Autodesk Inventor part; units mm, degrees
(part 4 of 9)
sketch "Sketch27" plane through (0, 0, 0) normal (1, 0, 0) x (0, 0, -1)
  circle A0 centre (0, 0) radius 14.2875
  circle A1 centre (-101.8395, -75.4579) radius 31.75
  line L0 (-136.8494, 13.4274) -> (-99.9912, -11.4177)
  line L1 (-99.9912, -11.4177) -> (-75.1461, 25.4405)
  line L2 (-75.1461, 25.4405) -> (-112.0043, 50.2856)
  line L3 (-112.0043, 50.2856) -> (-136.8494, 13.4274)
  line L4 (-136.8494, 13.4274) -> (-75.1461, 25.4405) construction
  line L5 (-99.9912, -11.4177) -> (-112.0043, 50.2856) construction
  circle A2 centre (-101.8395, -75.4579) radius 44.565
  circle A3 centre (0, 0) radius 15.915
  line L6 (-119.5903, -34.5807) -> (-6.3391, 14.598)
  line L7 (-67.9013, -104.3411) -> (12.12, -10.3147)
  circle A4 centre (0, 0) radius 47.752
  line L8 (-107.8805, 35.2378) -> (-5.6488, 47.4167)
  circle A5 centre (-105.9978, 19.434) radius 15.9156
  line L9 (-113.3646, 5.3259) -> (-22.1029, -42.3286)
  line L10 (-100.8674, 14.1953) -> (-107.9694, 12.3717)
  line L11 (-107.9694, 12.3717) -> (-113.0997, 17.6103)
  line L12 (-113.0997, 17.6103) -> (-111.1281, 24.6726)
  line L13 (-111.1281, 24.6726) -> (-104.0262, 26.4963)
  line L14 (-104.0262, 26.4963) -> (-98.8958, 21.2576)
  line L15 (-98.8958, 21.2576) -> (-100.8674, 14.1953)
  circle A6 centre (-105.9978, 19.434) radius 7.3323
  circle A7 centre (-101.8395, -75.4579) radius 9.5631
  circle A8 centre (-105.9978, 19.434) radius 9.5631
  circle A9 centre (-101.8395, -75.4579) radius 25.4
  circle A10 centre (-105.9978, 19.434) radius 25.4
  line L16 (-101.8395, -75.4579) -> (0, 0)
  circle A11 centre (0, 0) radius 50.8
  circle A12 centre (-105.9978, 19.434) radius 31.4309
  arc A13 (136.2027, -114.2876) -> (161.1415, 75.1415) centre (0, 0) ccw
  line L17 (0, 0) -> (136.2027, -114.2876)
  line L18 (0, 0) -> (173.2597, 0)
  circle A14 centre (33.8645, -135.5333) radius 88.9
  circle A15 centre (-76.4174, -178.6042) radius 25.4
  line L19 (-88.4199, -21.0451) -> (-93.4785, -9.396)
  circle A16 centre (-76.4174, -178.6042) radius 21.4859
  line L20 (-141.7593, -95.2683) -> (-95.6637, -188.1553)
  line L21 (-57.286, -74.4485) -> (-54.9371, -178.1175)
  line L22 (136.2027, -114.2876) -> (90.5518, -239.7125)
  circle A17 centre (31.6927, -141.5004) radius 88.9
  line L23 (-52.5492, -187.2916) -> (90.6599, -239.4154)
  line L24 (-105.9978, 19.434) -> (0, 0)
  line L25 (-76.4174, -204.0042) -> (-76.4174, -178.6042)
  line L26 (136.2027, -114.2876) -> (136.2027, -239.7125)
  line L27 (-58.8554, 19.434) -> (-105.9978, 19.434)
  circle A18 centre (-17.4502, -276.5193) radius 88.9
  line L28 (-501.4434, -455.6125) -> (248.5176, -455.6125)
  line L29 (-550.7161, -581.025) -> (328.0098, -581.025)
  circle A19 centre (-54.61, -366.7125) radius 88.9
  line L30 (-54.61, -280.9875) -> (-16.51, -280.9875)
  line L31 (-16.51, -280.9875) -> (-16.51, -363.5375)
  line L32 (-16.51, -363.5375) -> (-54.61, -363.5375)
  line L33 (-54.61, -363.5375) -> (-54.61, -280.9875)
  line L34 (-54.61, -322.2625) -> (-16.51, -322.2625)
  line L35 (-54.61, -366.7125) -> (-54.61, -277.8125)
  circle A20 centre (-16.51, -277.8125) radius 88.9
  line L36 (-16.51, -277.8125) -> (-16.51, -366.7125)
  circle A21 centre (-180.2765, -142.3655) radius 31.75
  circle A22 centre (-180.2765, -142.3655) radius 25.4
  circle A23 centre (-180.2765, -142.3655) radius 44.563
  circle A24 centre (-180.2765, -142.3655) radius 9.5631
  line L37 (-194.9575, -184.4408) -> (-91.0984, -220.6795)
  line L38 (-165.5955, -100.2902) -> (-61.7364, -136.5289)
  circle A25 centre (-76.4174, -178.6042) radius 44.563
  line L39 (-167.0299, -113.5109) -> (-119.1112, -9.1307)
  line L40 (-156.1209, -121.7605) -> (-135.7449, -104.3796)
  circle A26 centre (29.8359, -136.4768) radius 88.9
  line L41 (-116.4833, -117.4265) -> (-112.2994, -105.4355)
  line L42 (-85.3603, 16.259) -> (-85.3603, 6.734) projected
  arc A27 (-90.1228, 1.9715) -> (-85.3603, 6.734) centre (-90.1228, 6.734) ccw projected
  line L43 (-90.1228, 1.9715) -> (-121.8728, 1.9715) projected
  arc A28 (-126.6353, 6.734) -> (-121.8728, 1.9715) centre (-121.8728, 6.734) ccw projected
  line L44 (-126.6353, 6.734) -> (-126.6353, 16.259) projected
  line L45 (-126.6353, 16.259) -> (-132.3503, 16.259) projected
  arc A29 (-132.3503, 22.609) -> (-132.3503, 16.259) centre (-132.3503, 19.434) ccw projected
  line L46 (-132.3503, 22.609) -> (-126.6353, 22.609) projected
  line L47 (-126.6353, 22.609) -> (-126.6353, 32.134) projected
  arc A30 (-121.8728, 36.8965) -> (-126.6353, 32.134) centre (-121.8728, 32.134) ccw projected
  line L48 (-121.8728, 36.8965) -> (-90.1228, 36.8965) projected
  arc A31 (-85.3603, 32.134) -> (-90.1228, 36.8965) centre (-90.1228, 32.134) ccw projected
  line L49 (-85.3603, 32.134) -> (-85.3603, 22.609) projected
  line L50 (-85.3603, 22.609) -> (-79.6453, 22.609) projected
  arc A32 (-79.6453, 16.259) -> (-79.6453, 22.609) centre (-79.6453, 19.434) ccw projected
  line L51 (-79.6453, 16.259) -> (-85.3603, 16.259) projected
  circle A33 centre (-76.4174, -178.6042) radius 13.335 projected
  circle A34 centre (-187.1176, -166.8269) radius 2.4892 projected
  circle A35 centre (-174.2102, -166.8866) radius 2.4892 projected
  circle A36 centre (-167.2175, -120.5501) radius 2.4892 projected
  circle A37 centre (-180.1195, -116.9252) radius 2.4892 projected
  circle A38 centre (-193.0957, -120.1058) radius 2.4892 projected
  circle A39 centre (-186.8225, -117.6771) radius 2.4892 projected
  circle A40 centre (-173.4354, -117.9041) radius 2.4892 projected
  circle A41 centre (-168.1768, -164.3742) radius 2.4892 projected
  circle A42 centre (-180.6733, -167.7222) radius 2.4892 projected
  circle A43 centre (-193.0957, -164.2646) radius 2.4892 projected
  arc A44 (-177.4857, -133.2108) -> (-183.7867, -151.2692) centre (-180.6362, -142.24) ccw projected
  arc A45 (-183.3071, -151.4366) -> (-177.0061, -133.3781) centre (-180.1566, -142.4074) ccw projected
  circle A46 centre (-85.7798, -94.9817) radius 2.4892 projected
  circle A47 centre (-110.3931, -99.2933) radius 2.4892 projected
  circle A48 centre (-101.8395, -50.0579) radius 2.4892 projected
  circle A49 centre (-124.2369, -62.8574) radius 2.4892 projected
  circle A50 centre (-110.6604, -51.6228) radius 2.4892 projected
  circle A51 centre (-93.2858, -99.3592) radius 2.4892 projected
  circle A52 centre (-118.4334, -56.0666) radius 2.4892 projected
  circle A53 centre (-93.0185, -51.5569) radius 2.4892 projected
  circle A54 centre (-101.8395, -100.8579) radius 2.4892 projected
  circle A55 centre (-80.2428, -88.2574) radius 2.4892 projected
  arc A56 (-99.4903, -84.728) -> (-104.0551, -66.155) centre (-101.7058, -75.4251) ccw projected
  arc A57 (-99.6119, -84.758) -> (-99.4903, -84.728) centre (-101.8395, -75.4579) ccw projected
  arc A58 (-99.7334, -84.7881) -> (-99.6119, -84.758) centre (-101.9731, -75.491) ccw projected
  arc A59 (-99.8547, -84.8183) -> (-99.7334, -84.7881) centre (-102.1066, -75.5241) ccw projected
  arc A60 (-104.4917, -66.2632) -> (-99.8547, -84.8183) centre (-102.2399, -75.5574) ccw projected
  arc A61 (-104.3463, -66.227) -> (-104.4917, -66.2632) centre (-102.1066, -75.5241) ccw projected
  arc A62 (-104.2008, -66.1909) -> (-104.3463, -66.227) centre (-101.9731, -75.491) ccw projected
  arc A63 (-104.0551, -66.155) -> (-104.2008, -66.1909) centre (-101.8395, -75.4579) ccw projected
  circle A64 centre (239.2356, -31.496) radius 3.3782 projected
  circle A65 centre (223.7295, 90.3926) radius 3.3782 projected
  circle A66 centre (239.2356, 31.496) radius 3.3782 projected
  circle A67 centre (221.404, -95.9477) radius 3.3782 projected
  line L52 (-35.2916, -50.8) -> (42.0514, -50.8) projected
  arc A68 (74.705, -62.6849) -> (42.0514, -50.8) centre (42.0514, -101.6) ccw projected
  line L53 (74.705, -62.6849) -> (143.4787, -120.3929) projected
  arc A69 (143.8351, -124.9069) -> (143.4787, -120.3929) centre (141.4378, -122.8251) ccw projected
  arc A70 (141.8978, -127.1034) -> (143.8351, -124.9069) centre (0, 0) ccw projected
  arc A71 (141.8978, -127.1034) -> (141.494, -128.2246) centre (143.0803, -128.1626) ccw projected
  line L54 (141.6194, -131.4328) -> (141.494, -128.2246) projected
  arc A72 (141.6194, -131.4328) -> (142.123, -132.5318) centre (143.2057, -131.3708) ccw projected
  line L55 (142.123, -132.5318) -> (176.2311, -164.3381) projected
  arc A73 (176.2311, -164.3381) -> (194.6236, -163.2104) centre (184.8924, -155.0499) ccw projected
  arc A74 (194.6236, -163.2104) -> (235.5329, 95.0804) centre (0, 0) ccw projected
  arc A75 (235.5329, 95.0804) -> (218.389, 101.8364) centre (223.7562, 90.3263) ccw projected
  line L56 (218.389, 101.8364) -> (173.6183, 80.9596) projected
  arc A76 (152.1493, 76.2) -> (173.6183, 80.9596) centre (152.1493, 127) ccw projected
  line L57 (152.1493, 76.2) -> (-101.6, 76.2) projected
  line L58 (-101.6, 76.2) -> (-199.482, -21.682) projected
  line L59 (-199.482, -21.682) -> (-199.482, -255.599) projected
  line L60 (-199.482, -255.599) -> (-35.2916, -255.599) projected
  line L61 (-35.2916, -255.599) -> (-35.2916, -50.8) projected
  line L62 (149.831, -89.2272) -> (89.9434, -38.9755) projected
  arc A77 (88.9, -36.7379) -> (89.9434, -38.9755) centre (91.821, -36.7379) ccw projected
  line L63 (88.9, -36.7379) -> (88.9, -15.621) projected
  arc A78 (91.821, -12.7) -> (88.9, -15.621) centre (91.821, -15.621) ccw projected
  line L64 (91.821, -12.7) -> (174.1799, -12.7) projected
  arc A79 (177.0893, -15.8819) -> (174.1799, -12.7) centre (174.1799, -15.621) ccw projected
  arc A80 (154.2425, -88.4425) -> (177.0893, -15.8819) centre (0, 0) ccw projected
  arc A81 (149.831, -89.2272) -> (154.2425, -88.4425) centre (151.7086, -86.9895) ccw projected
  line L65 (88.9, -0.254) -> (88.9, 0.254) projected
  arc A82 (91.821, 3.175) -> (88.9, 0.254) centre (91.821, 0.254) ccw projected
  line L66 (91.821, 3.175) -> (174.4218, 3.175) projected
  arc A83 (177.3428, 0.254) -> (174.4218, 3.175) centre (174.4218, 0.254) ccw projected
  line L67 (177.3428, 0.254) -> (177.3428, -0.254) projected
  arc A84 (174.4218, -3.175) -> (177.3428, -0.254) centre (174.4218, -0.254) ccw projected
  line L68 (174.4218, -3.175) -> (91.821, -3.175) projected
  arc A85 (88.9, -0.254) -> (91.821, -3.175) centre (91.821, -0.254) ccw projected
  arc A86 (177.0893, 15.8819) -> (169.6939, 53.0738) centre (0, 0) ccw projected
  arc A87 (174.1799, 12.7) -> (177.0893, 15.8819) centre (174.1799, 15.621) ccw projected
  line L69 (174.1799, 12.7) -> (91.821, 12.7) projected
  arc A88 (88.9, 15.621) -> (91.821, 12.7) centre (91.821, 15.621) ccw projected
  line L70 (88.9, 15.621) -> (88.9, 17.1891) projected
  arc A89 (90.5865, 19.8364) -> (88.9, 17.1891) centre (91.821, 17.1891) ccw projected
  line L71 (90.5865, 19.8364) -> (165.6716, 54.8492) projected
  arc A90 (169.6939, 53.0738) -> (165.6716, 54.8492) centre (166.9061, 52.2019) ccw projected
  arc A91 (180.8991, -105.7674) -> (203.0448, 51.8076) centre (0, 0) ccw projected
  arc A92 (204.8485, 54.889) -> (203.0448, 51.8076) centre (205.5059, 52.4355) ccw projected
  line L72 (204.8485, 54.889) -> (206.0753, 55.2177) projected
  arc A93 (209.1938, 53.3924) -> (206.0753, 55.2177) centre (206.7327, 52.7643) ccw projected
  arc A94 (186.3731, -108.9857) -> (209.1938, 53.3924) centre (0, 0) ccw projected
  arc A95 (182.8723, -109.8807) -> (186.3731, -108.9857) centre (184.1805, -107.7035) ccw projected
  line L73 (182.8723, -109.8807) -> (181.7836, -109.2266) projected
  arc A96 (180.8991, -105.7674) -> (181.7836, -109.2266) centre (183.0918, -107.0494) ccw projected
  arc A97 (159.1231, -92.6879) -> (178.5072, 45.237) centre (0, 0) ccw projected
  arc A98 (180.312, 48.3145) -> (178.5072, 45.237) centre (180.9694, 45.861) ccw projected
  line L74 (180.312, 48.3145) -> (181.5388, 48.6432) projected
  arc A99 (184.6584, 46.8139) -> (181.5388, 48.6432) centre (182.1962, 46.1897) ccw projected
  arc A100 (164.6013, -95.8992) -> (184.6584, 46.8139) centre (0, 0) ccw projected
  arc A101 (161.0985, -96.7977) -> (164.6013, -95.8992) centre (162.4067, -94.6205) ccw projected
  line L75 (161.0985, -96.7977) -> (160.0098, -96.1436) projected
  arc A102 (159.1231, -92.6879) -> (160.0098, -96.1436) centre (161.3179, -93.9664) ccw projected
  line L76 (171.9854, -103.3393) -> (170.8967, -102.6851) projected
  arc A103 (170.0112, -99.2275) -> (170.8967, -102.6851) centre (172.2049, -100.5079) ccw projected
  arc A104 (170.0112, -99.2275) -> (190.7761, 48.5222) centre (0, 0) ccw projected
  arc A105 (192.5803, 51.6017) -> (190.7761, 48.5222) centre (193.2377, 49.1483) ccw projected
  line L77 (192.5803, 51.6017) -> (193.8071, 51.9305) projected
  arc A106 (196.9261, 50.1033) -> (193.8071, 51.9305) centre (194.4645, 49.477) ccw projected
  arc A107 (175.4872, -102.4426) -> (196.9261, 50.1033) centre (0, 0) ccw projected
  arc A108 (171.9854, -103.3393) -> (175.4872, -102.4426) centre (173.2936, -101.1621) ccw projected
  circle A109 centre (187.962, 68.4126) radius 2.5527 projected
  circle A110 centre (160.7915, -118.9794) radius 2.5527 projected
  circle A111 centre (0, 0) radius 13.335 projected
  line L78 (-177.4857, -133.2108) -> (-177.0061, -133.3781) projected
  line L79 (-183.3071, -151.4366) -> (-183.7867, -151.2692) projected
  point P0 (-35.56, -322.2625)
  dimension "d821" = 63.5
  dimension "d820" = 28.575
  dimension "d822" = 44.45
  dimension "d823" = 31.83
  dimension "d824" = 89.13
  dimension "d825" = 95.504
  dimension "d826" = 31.8313
  dimension "d827" = 12.7
  dimension "d828" = 19.1262
  dimension "d829" = 19.1262
  dimension "d830" = 50.8
  dimension "d831" = 50.8
  dimension "d832" = 107.7646
  dimension "d833" = 126.7485
  dimension "d834" = 101.6
  dimension "d835" = 127
  dimension "d836" = 40
  dimension "d837" = 177.8
  dimension "d838" = 50.8
  dimension "d839" = 12.7
  dimension "d840" = 6.35
  dimension "d841" = 106.233
  dimension "d842" = 152.4
  dimension "d843" = 279.1458
  dimension "d844" = 25
  dimension "d845" = 20
  dimension "d846" = 47.1424
  dimension "d847" = 42.9717
  dimension "d848" = 125.4125
  dimension "d849" = 656.1665
  dimension "d850" = 82.55
  dimension "d851" = 38.1
  dimension "d852" = 1.5989
  dimension "d853" = 35.56
  dimension "d854" = 215.9
  dimension "d855" = 215.9
  dimension "d856" = 26.7819
  dimension "d857" = 114.8539
  dimension "d858" = 109.9998
  dimension "d859" = 581.025
  dimension "d860" = 455.6125
  dimension "d861" = 12.7
  dimension "d862" = 89.1261
  constraints: 84 end point, 26 point on circle, 24 tangent, 23 centre point, 19 coincident, 9 midpoint, 7 perpendicular, 6 equal radius, 6 horizontal, 6 line through centre, 6 point on line, 4 parallel, 4 vertical, 3 concentric, 2 vertical alignment, 26 other
  measures "d820" diameter of A0
  measures "d822" distance of L0.end L1.end
  measures "d823" diameter of A3
  measures "d824" diameter of A2
  measures "d825" diameter of A4
  measures "d826" diameter of A5
  measures "d827" distance between parallel lines of L14 L11
  measures "d828" diameter of A7
  measures "d829" diameter of A8
  measures "d830" diameter of A9
  measures "d831" diameter of A10
  measures "d832" distance of A0.centre point (-105.998, 19.434)
  measures "d833" distance of point (0, 0) point (-101.84, -75.458)
  measures "d834" diameter of A11
  measures "d835" radial gap between concentric circles of A13 A11
  measures "d836" angle of L18 L17
  measures "d837" diameter of A14
  measures "d838" diameter of A15
  measures "d839" distance of L19.start L19.end
  measures "d840" distance of A17.centre A14.centre
  measures "d841" distance of point (-101.84, -75.458) A15.centre
  measures "d842" distance of L23.start L23.end
  measures "d843" vertical distance of L25.start A13.end
  measures "d845" angle of L26 L22
  measures "d846" distance of point (-105.998, 19.434) L27.start
  measures "d847" diameter of A16
  measures "d848" distance between parallel lines of L28 L29
  measures "d849" distance from line of A13.end L29
  measures "d850" distance of L33.start L30.start
  measures "d851" distance of L31.end L33.start
  measures "d852" distance of L36.start A18.centre
  measures "d853" horizontal distance of A11.centre point (-35.56, -322.262)
  measures "d854" distance from line of L28 L26.end
  measures "d855" distance from line of L28 L22.end
  measures "d856" distance of L40.start L40.end
  measures "d857" distance of L39.start L39.end
  measures "d858" distance of A21.centre L25.end
  measures "d859" distance from line of L29 point (0, 0)
  measures "d860" distance from line of L28 L17.start
  measures "d861" distance of L41.start L41.end
  measures "d862" diameter of A23
hole "Hole10" at (0, 19.434, 58.8554) direction (-1, 0, 0) diameter 4.9784 end through all clearance for "Flat Head Machine Screw (82)" size "#10" standard "Ansi Unified Screw Threads"
sketch "Sketch28" plane through (0, 0, 0) normal (1, 0, 0) x (0, 0, -1)
  line L0 (-85.3603, 16.259) -> (-85.3603, 6.734) projected
  arc A0 (-90.1228, 1.9715) -> (-85.3603, 6.734) centre (-90.1228, 6.734) ccw projected
  line L1 (-90.1228, 1.9715) -> (-121.8728, 1.9715) projected
  arc A1 (-126.6353, 6.734) -> (-121.8728, 1.9715) centre (-121.8728, 6.734) ccw projected
  line L2 (-126.6353, 6.734) -> (-126.6353, 16.259) projected
  line L3 (-126.6353, 16.259) -> (-132.3503, 16.259) projected
  arc A2 (-132.3503, 22.609) -> (-132.3503, 16.259) centre (-132.3503, 19.434) ccw projected
  line L4 (-132.3503, 22.609) -> (-126.6353, 22.609) projected
  line L5 (-126.6353, 22.609) -> (-126.6353, 32.134) projected
  arc A3 (-121.8728, 36.8965) -> (-126.6353, 32.134) centre (-121.8728, 32.134) ccw projected
  line L6 (-121.8728, 36.8965) -> (-90.1228, 36.8965) projected
  arc A4 (-85.3603, 32.134) -> (-90.1228, 36.8965) centre (-90.1228, 32.134) ccw projected
  line L7 (-85.3603, 32.134) -> (-85.3603, 22.609) projected
  line L8 (-85.3603, 22.609) -> (-79.6453, 22.609) projected
  arc A5 (-79.6453, 16.259) -> (-79.6453, 22.609) centre (-79.6453, 19.434) ccw projected
  line L9 (-79.6453, 16.259) -> (-85.3603, 16.259) projected
  circle A6 centre (-187.1176, -166.8269) radius 2.4892 projected
  circle A7 centre (-174.2102, -166.8866) radius 2.4892 projected
  circle A8 centre (-167.2175, -120.5501) radius 2.4892 projected
  circle A9 centre (-180.1195, -116.9252) radius 2.4892 projected
  circle A10 centre (-193.0957, -120.1058) radius 2.4892 projected
  circle A11 centre (-186.8225, -117.6771) radius 2.4892 projected
  circle A12 centre (-173.4354, -117.9041) radius 2.4892 projected
  circle A13 centre (-168.1768, -164.3742) radius 2.4892 projected
  circle A14 centre (-180.6733, -167.7222) radius 2.4892 projected
  circle A15 centre (-193.0957, -164.2646) radius 2.4892 projected
  circle A16 centre (0, 0) radius 13.335 projected
  circle A17 centre (160.7915, -118.9794) radius 2.5527 projected
  line L10 (182.8723, -109.8807) -> (181.7836, -109.2266) projected
  arc A18 (170.0112, -99.2275) -> (190.7761, 48.5222) centre (0, 0) ccw projected
  line L11 (204.8485, 54.889) -> (206.0753, 55.2177) projected
  arc A19 (175.4872, -102.4426) -> (196.9261, 50.1033) centre (0, 0) ccw projected
  arc A20 (159.1231, -92.6879) -> (178.5072, 45.237) centre (0, 0) ccw projected
  line L12 (180.312, 48.3145) -> (181.5388, 48.6432) projected
  arc A21 (164.6013, -95.8992) -> (184.6584, 46.8139) centre (0, 0) ccw projected
  line L13 (161.0985, -96.7977) -> (160.0098, -96.1436) projected
  arc A22 (180.8991, -105.7674) -> (203.0448, 51.8076) centre (0, 0) ccw projected
  line L14 (192.5803, 51.6017) -> (193.8071, 51.9305) projected
  arc A23 (186.3731, -108.9857) -> (209.1938, 53.3924) centre (0, 0) ccw projected
  line L15 (171.9854, -103.3393) -> (170.8967, -102.6851) projected
  circle A24 centre (239.2356, -31.496) radius 3.3782 projected
  circle A25 centre (223.7295, 90.3926) radius 3.3782 projected
  circle A26 centre (239.2356, 31.496) radius 3.3782 projected
  circle A27 centre (221.404, -95.9477) radius 3.3782 projected
  line L16 (-35.2916, -50.8) -> (42.0514, -50.8) projected
  arc A28 (74.705, -62.6849) -> (42.0514, -50.8) centre (42.0514, -101.6) ccw projected
  line L17 (74.705, -62.6849) -> (143.4787, -120.3929) projected
  arc A29 (143.8351, -124.9069) -> (143.4787, -120.3929) centre (141.4378, -122.8251) ccw projected
  arc A30 (141.8978, -127.1034) -> (143.8351, -124.9069) centre (0, 0) ccw projected
  arc A31 (141.8978, -127.1034) -> (141.494, -128.2246) centre (143.0803, -128.1626) ccw projected
  line L18 (141.6194, -131.4328) -> (141.494, -128.2246) projected
  arc A32 (141.6194, -131.4328) -> (142.123, -132.5318) centre (143.2057, -131.3708) ccw projected
  line L19 (142.123, -132.5318) -> (176.2311, -164.3381) projected
  arc A33 (176.2311, -164.3381) -> (194.6236, -163.2104) centre (184.8924, -155.0499) ccw projected
  arc A34 (194.6236, -163.2104) -> (235.5329, 95.0804) centre (0, 0) ccw projected
  arc A35 (235.5329, 95.0804) -> (218.389, 101.8364) centre (223.7562, 90.3263) ccw projected
  line L20 (218.389, 101.8364) -> (173.6183, 80.9596) projected
  arc A36 (152.1493, 76.2) -> (173.6183, 80.9596) centre (152.1493, 127) ccw projected
  line L21 (152.1493, 76.2) -> (-101.6, 76.2) projected
  line L22 (-101.6, 76.2) -> (-199.482, -21.682) projected
  line L23 (-199.482, -21.682) -> (-199.482, -255.599) projected
  line L24 (-199.482, -255.599) -> (-35.2916, -255.599) projected
  line L25 (-35.2916, -255.599) -> (-35.2916, -50.8) projected
  line L26 (149.831, -89.2272) -> (89.9434, -38.9755) projected
  line L27 (88.9, -36.7379) -> (88.9, -15.621) projected
  line L28 (91.821, -12.7) -> (174.1799, -12.7) projected
  arc A37 (154.2425, -88.4425) -> (177.0893, -15.8819) centre (0, 0) ccw projected
  line L29 (88.9, -0.254) -> (88.9, 0.254) projected
  line L30 (91.821, 3.175) -> (174.4218, 3.175) projected
  line L31 (177.3428, 0.254) -> (177.3428, -0.254) projected
  line L32 (174.4218, -3.175) -> (91.821, -3.175) projected
  arc A38 (177.0893, 15.8819) -> (169.6939, 53.0738) centre (0, 0) ccw projected
  line L33 (174.1799, 12.7) -> (91.821, 12.7) projected
  line L34 (88.9, 15.621) -> (88.9, 17.1891) projected
  line L35 (90.5865, 19.8364) -> (165.6716, 54.8492) projected
  circle A39 centre (-80.2428, -88.2574) radius 2.4892 projected
  circle A40 centre (-101.8395, -100.8579) radius 2.4892 projected
  circle A41 centre (-93.0185, -51.5569) radius 2.4892 projected
  circle A42 centre (-93.2858, -99.3592) radius 2.4892 projected
  circle A43 centre (-110.6604, -51.6228) radius 2.4892 projected
  circle A44 centre (-124.2369, -62.8574) radius 2.4892 projected
  circle A45 centre (-101.8395, -50.0579) radius 2.4892 projected
  circle A46 centre (-110.3931, -99.2933) radius 2.4892 projected
  circle A47 centre (-85.7798, -94.9817) radius 2.4892 projected
  line L36 (-121.8728, 6.734) -> (-90.1228, 6.734)
  line L37 (-90.1228, 6.734) -> (-90.1228, 32.134)
  line L38 (-90.1228, 32.134) -> (-121.8728, 32.134)
  line L39 (-121.8728, 32.134) -> (-121.8728, 6.734)
  line L40 (-121.8728, 6.734) -> (-90.1228, 32.134) construction
  line L41 (-90.1228, 6.734) -> (-121.8728, 32.134) construction
  line L42 (-131.3978, 57.3308) -> (-80.5978, 57.3308)
  line L43 (-105.9978, 19.434) -> (-105.9978, 57.3308)
  line L44 (-105.9978, -16.3292) -> (-105.9978, 19.434)
  line L45 (-112.3478, -16.3292) -> (-99.6478, -16.3292)
  circle A48 centre (-112.3478, -16.3292) radius 2.5527
  circle A49 centre (-99.6478, -16.3292) radius 2.5527
  circle A50 centre (-80.5978, 57.3308) radius 2.5527
  circle A51 centre (-131.3978, 57.3308) radius 2.5527
  line L46 (-112.3478, -13.7765) -> (-99.6478, -13.7765)
  line L47 (-99.6478, -18.8819) -> (-112.3478, -18.8819)
  line L48 (-131.3978, 59.8835) -> (-80.5978, 59.8835)
  line L49 (-80.5978, 54.7781) -> (-131.3978, 54.7781)
  arc A52 (174.1799, 12.7) -> (177.0893, 15.8819) centre (174.1799, 15.621) ccw projected
  arc A53 (88.9, 15.621) -> (91.821, 12.7) centre (91.821, 15.621) ccw projected
  arc A54 (90.5865, 19.8364) -> (88.9, 17.1891) centre (91.821, 17.1891) ccw projected
  arc A55 (169.6939, 53.0738) -> (165.6716, 54.8492) centre (166.9061, 52.2019) ccw projected
  arc A56 (91.821, 3.175) -> (88.9, 0.254) centre (91.821, 0.254) ccw projected
  arc A57 (177.3428, 0.254) -> (174.4218, 3.175) centre (174.4218, 0.254) ccw projected
  arc A58 (174.4218, -3.175) -> (177.3428, -0.254) centre (174.4218, -0.254) ccw projected
  arc A59 (88.9, -0.254) -> (91.821, -3.175) centre (91.821, -0.254) ccw projected
  arc A60 (88.9, -36.7379) -> (89.9434, -38.9755) centre (91.821, -36.7379) ccw projected
  arc A61 (91.821, -12.7) -> (88.9, -15.621) centre (91.821, -15.621) ccw projected
  arc A62 (177.0893, -15.8819) -> (174.1799, -12.7) centre (174.1799, -15.621) ccw projected
  arc A63 (149.831, -89.2272) -> (154.2425, -88.4425) centre (151.7086, -86.9895) ccw projected
  arc A64 (170.0112, -99.2275) -> (170.8967, -102.6851) centre (172.2049, -100.5079) ccw projected
  arc A65 (192.5803, 51.6017) -> (190.7761, 48.5222) centre (193.2377, 49.1483) ccw projected
  arc A66 (196.9261, 50.1033) -> (193.8071, 51.9305) centre (194.4645, 49.477) ccw projected
  arc A67 (171.9854, -103.3393) -> (175.4872, -102.4426) centre (173.2936, -101.1621) ccw projected
  arc A68 (180.312, 48.3145) -> (178.5072, 45.237) centre (180.9694, 45.861) ccw projected
  arc A69 (184.6584, 46.8139) -> (181.5388, 48.6432) centre (182.1962, 46.1897) ccw projected
  arc A70 (161.0985, -96.7977) -> (164.6013, -95.8992) centre (162.4067, -94.6205) ccw projected
  arc A71 (159.1231, -92.6879) -> (160.0098, -96.1436) centre (161.3179, -93.9664) ccw projected
  arc A72 (204.8485, 54.889) -> (203.0448, 51.8076) centre (205.5059, 52.4355) ccw projected
  arc A73 (209.1938, 53.3924) -> (206.0753, 55.2177) centre (206.7327, 52.7643) ccw projected
  arc A74 (182.8723, -109.8807) -> (186.3731, -108.9857) centre (184.1805, -107.7035) ccw projected
  arc A75 (180.8991, -105.7674) -> (181.7836, -109.2266) centre (183.0918, -107.0494) ccw projected
  arc A76 (-99.6119, -84.758) -> (-99.4903, -84.728) centre (-101.8395, -75.4579) ccw projected
  arc A77 (-99.4903, -84.728) -> (-104.0551, -66.155) centre (-101.7058, -75.4251) ccw projected
  arc A78 (-99.7334, -84.7881) -> (-99.6119, -84.758) centre (-101.9731, -75.491) ccw projected
  arc A79 (-99.8547, -84.8183) -> (-99.7334, -84.7881) centre (-102.1066, -75.5241) ccw projected
  arc A80 (-104.4917, -66.2632) -> (-99.8547, -84.8183) centre (-102.2399, -75.5574) ccw projected
  arc A81 (-104.3463, -66.227) -> (-104.4917, -66.2632) centre (-102.1066, -75.5241) ccw projected
  arc A82 (-104.2008, -66.1909) -> (-104.3463, -66.227) centre (-101.9731, -75.491) ccw projected
  arc A83 (-104.0551, -66.155) -> (-104.2008, -66.1909) centre (-101.8395, -75.4579) ccw projected
  point P0 (-105.9978, 19.434)
  dimension "d478" = 50.8
  dimension "d479" = 12.7
  dimension "d480" = 5.1054
  dimension "d554" = 35.7632
  dimension "d555" = 37.8968
  constraints: 28 end point, 8 midpoint, 8 point on circle, 7 tangent, 6 coincident, 4 centre point, 4 horizontal, 3 equal radius, 2 parallel, 2 vertical, 1 perpendicular, 1 point on line
  measures "d478" distance of L42.end L42.start
  measures "d479" distance of L45.start L45.end
  measures "d480" diameter of A48
  measures "d554" distance from line of point (-105.998, 19.434) L45
  measures "d555" distance from line of L43.start L42
extrude "Extrusion17" cut sketch "Sketch28" against normal blind 25.4 contours L49 A51 L42 L22 | L22 L42 L43 L49 | L42 A51 L48 L22 | L22 L48 A50 L42 | L43 L42 A50 L49 | A51 | A50 | L45 A48 L46 L44 | L45 A49 L47 A48 | L44 L46 A49 L45 | A48 | A49
sketch "Sketch29" plane through (0, 0, 0) normal (1, 0, 0) x (0, 0, -1)
  arc A0 (194.6236, -163.2104) -> (235.5329, 95.0804) centre (0, 0) ccw projected
  line L0 (-199.482, -255.599) -> (-35.2916, -255.599) projected
  arc A1 (141.8978, -127.1034) -> (143.8351, -124.9069) centre (0, 0) ccw projected
  line L1 (74.705, -62.6849) -> (143.4787, -120.3929) projected
  line L2 (-35.2916, -255.599) -> (-35.2916, -50.8) projected
  line L3 (-35.2916, -255.599) -> (-35.2916, -230.199)
  line L4 (72.1517, -230.199) -> (-35.2916, -230.199)
  line L5 (142.123, -132.5318) -> (176.2311, -164.3381) projected
  line L6 (141.6194, -131.4328) -> (141.494, -128.2246) projected
  line L7 (-35.2916, -255.599) -> (149.8274, -255.599)
  line L8 (87.0583, -242.899) -> (183.6323, -242.899) construction
  circle A2 centre (145.0649, -113.4346) radius 6.35 construction
  line L9 (145.0649, -113.4346) -> (145.0649, -320.5339) construction
  line L10 (145.0649, -113.4346) -> (118.5854, -263.6072) construction
  line L11 (145.0649, -113.4346) -> (83.6885, -282.0649) construction
  line L12 (145.0649, -113.4346) -> (54.5486, -270.2133) construction
  arc A3 (154.2425, -88.4425) -> (177.0893, -15.8819) centre (0, 0) ccw construction
  line L13 (114.3, -157.1959) -> (114.3, -116.9566)
  arc A4 (176.2311, -164.3381) -> (194.6236, -163.2104) centre (184.8924, -155.0499) ccw construction
  line L14 (88.9, -36.7379) -> (88.9, -15.621) projected
  line L15 (149.8274, -255.599) -> (194.6236, -163.2104)
  line L16 (114.3, -157.1959) -> (72.1517, -230.199)
  line L17 (114.3, -116.9566) -> (179.2278, -123.3639)
  line L18 (179.2278, -123.3639) -> (194.6236, -163.2104)
  circle A5 centre (160.7915, -118.9794) radius 2.5527 projected
  arc A6 (143.8351, -124.9069) -> (143.4787, -120.3929) centre (141.4378, -122.8251) ccw projected
  point P0 (165.389, -138.7778)
  point P1 (102.5661, -230.199)
  point P2 (70.3186, -242.899)
  point P3 (97.9437, -242.899)
  point P4 (122.2368, -242.899)
  point P5 (145.0649, -242.899)
  point P6 (177.3458, -12.7)
  point P7 (152.4791, -91.4492)
  point P8 (184.8924, -167.7499)
  dimension "d495" = 25.4
  dimension "d497" = 12.7
  dimension "d498" = 12.7
  dimension "d499" = 10
  dimension "d501" = 20
  dimension "d502" = 30
  dimension "d507" = 4.7625
  dimension "d508" = 25.4
  dimension "d516" = 4.7625
  constraints: 26 end point, 9 point on line, 4 tangent, 2 coincident, 2 horizontal, 2 parallel, 1 centre point, 1 collinear, 1 point on circle, 1 vertical
  measures "d495" distance between parallel lines of L4 L7
  measures "d497" distance between parallel lines of L7 L8
  measures "d498" diameter of A2
  measures "d499" angle of L10 L9
  measures "d501" angle of L9 L11
  measures "d502" angle of L9 L12
  measures "d507" horizontal distance of L7.end point (145.065, -242.899)
  measures "d508" distance between parallel lines of L13 L14
  measures "d516" distance between parallel lines of L16 L12
extrude "Extrusion18" add sketch "Sketch29" against normal up to surface (3.175 mm away) contours L2 L4 L16 L13 L17 L18 L15 L7
fillet "Fillet7" radius 3.175 5 edges at (-1.5875, -157.1959, -114.3) (-1.5875, -230.199, -72.1517) (-1.5875, -230.199, 35.2916) (-1.5875, -50.8, 35.2916) (-1.5875, -163.2104, -194.6236)
hole "ChuteHoles" at (0, -242.899, -70.3186) at (0, -242.899, -97.9437) at (0, -242.899, -122.2368) at (0, -242.899, -145.0649) at (0, -113.4346, -145.0649) direction (-1, 0, 0) diameter 5.1054 end through all clearance for "Flat Head Machine Screw (82)" size "#10" standard "Ansi Unified Screw Threads"
sketch "Sketch32" plane through (0, 0, 0) normal (1, 0, 0) x (0, 0, -1)
  line L0 (152.1493, 76.2) -> (-101.6, 76.2) projected
  line L1 (-199.482, -255.599) -> (149.8274, -255.599) projected
  line L2 (-199.482, -21.682) -> (-199.482, -255.599) projected
  circle A0 centre (145.0649, -242.899) radius 2.5527 projected
  circle A1 centre (97.9437, -242.899) radius 2.5527 projected
  circle A2 centre (70.3186, -242.899) radius 2.5527 projected
  circle A3 centre (122.2368, -242.899) radius 2.5527 projected
  circle A4 centre (145.0649, -113.4346) radius 2.5527 projected
  line L3 (-35.2916, -227.024) -> (-35.2916, -53.975) projected
  arc A5 (-32.1166, -50.8) -> (-35.2916, -53.975) centre (-32.1166, -53.975) ccw projected
  line L4 (-32.1166, -50.8) -> (42.0514, -50.8) projected
  arc A6 (74.705, -62.6849) -> (42.0514, -50.8) centre (42.0514, -101.6) ccw projected
  line L5 (74.705, -62.6849) -> (142.7266, -119.7618) projected
  line L6 (114.3, -116.9566) -> (142.7266, -119.7618) projected
  line L7 (114.3, -156.3452) -> (114.3, -116.9566) projected
  arc A7 (113.8746, -157.9327) -> (114.3, -156.3452) centre (111.125, -156.3452) ccw projected
  line L8 (73.0682, -228.6115) -> (113.8746, -157.9327) projected
  arc A8 (70.3186, -230.199) -> (73.0682, -228.6115) centre (70.3186, -227.024) ccw projected
  line L9 (-32.1166, -230.199) -> (70.3186, -230.199) projected
  arc A9 (-35.2916, -227.024) -> (-32.1166, -230.199) centre (-32.1166, -227.024) ccw projected
  circle A10 centre (160.7915, -118.9794) radius 2.5527 projected
  circle A11 centre (0, 0) radius 13.335 projected
  circle A12 centre (187.962, 68.4126) radius 2.5527 projected
  line L10 (171.9854, -103.3393) -> (170.8967, -102.6851) projected
  arc A13 (170.0112, -99.2275) -> (170.8967, -102.6851) centre (172.2049, -100.5079) ccw projected
  arc A14 (170.0112, -99.2275) -> (190.7761, 48.5222) centre (0, 0) ccw projected
  arc A15 (192.5803, 51.6017) -> (190.7761, 48.5222) centre (193.2377, 49.1483) ccw projected
  line L11 (192.5803, 51.6017) -> (193.8071, 51.9305) projected
  arc A16 (196.9261, 50.1033) -> (193.8071, 51.9305) centre (194.4645, 49.477) ccw projected
  arc A17 (175.4872, -102.4426) -> (196.9261, 50.1033) centre (0, 0) ccw projected
  arc A18 (171.9854, -103.3393) -> (175.4872, -102.4426) centre (173.2936, -101.1621) ccw projected
  arc A19 (159.1231, -92.6879) -> (178.5072, 45.237) centre (0, 0) ccw projected
  arc A20 (180.312, 48.3145) -> (178.5072, 45.237) centre (180.9694, 45.861) ccw projected
  line L12 (180.312, 48.3145) -> (181.5388, 48.6432) projected
  arc A21 (184.6584, 46.8139) -> (181.5388, 48.6432) centre (182.1962, 46.1897) ccw projected
  arc A22 (164.6013, -95.8992) -> (184.6584, 46.8139) centre (0, 0) ccw projected
  arc A23 (161.0985, -96.7977) -> (164.6013, -95.8992) centre (162.4067, -94.6205) ccw projected
  line L13 (161.0985, -96.7977) -> (160.0098, -96.1436) projected
  arc A24 (159.1231, -92.6879) -> (160.0098, -96.1436) centre (161.3179, -93.9664) ccw projected
  arc A25 (180.8991, -105.7674) -> (203.0448, 51.8076) centre (0, 0) ccw projected
  arc A26 (204.8485, 54.889) -> (203.0448, 51.8076) centre (205.5059, 52.4355) ccw projected
  line L14 (204.8485, 54.889) -> (206.0753, 55.2177) projected
  arc A27 (209.1938, 53.3924) -> (206.0753, 55.2177) centre (206.7327, 52.7643) ccw projected
  arc A28 (186.3731, -108.9857) -> (209.1938, 53.3924) centre (0, 0) ccw projected
  arc A29 (182.8723, -109.8807) -> (186.3731, -108.9857) centre (184.1805, -107.7035) ccw projected
  line L15 (182.8723, -109.8807) -> (181.7836, -109.2266) projected
  arc A30 (180.8991, -105.7674) -> (181.7836, -109.2266) centre (183.0918, -107.0494) ccw projected
  arc A31 (177.0893, 15.8819) -> (169.6939, 53.0738) centre (0, 0) ccw projected
  arc A32 (174.1799, 12.7) -> (177.0893, 15.8819) centre (174.1799, 15.621) ccw projected
  line L16 (174.1799, 12.7) -> (91.821, 12.7) projected
  arc A33 (88.9, 15.621) -> (91.821, 12.7) centre (91.821, 15.621) ccw projected
  line L17 (88.9, 15.621) -> (88.9, 17.1891) projected
  arc A34 (90.5865, 19.8364) -> (88.9, 17.1891) centre (91.821, 17.1891) ccw projected
  line L18 (90.5865, 19.8364) -> (165.6716, 54.8492) projected
  arc A35 (169.6939, 53.0738) -> (165.6716, 54.8492) centre (166.9061, 52.2019) ccw projected
  line L19 (88.9, -0.254) -> (88.9, 0.254) projected
  arc A36 (91.821, 3.175) -> (88.9, 0.254) centre (91.821, 0.254) ccw projected
  line L20 (91.821, 3.175) -> (174.4218, 3.175) projected
  arc A37 (177.3428, 0.254) -> (174.4218, 3.175) centre (174.4218, 0.254) ccw projected
  line L21 (177.3428, 0.254) -> (177.3428, -0.254) projected
  arc A38 (174.4218, -3.175) -> (177.3428, -0.254) centre (174.4218, -0.254) ccw projected
  line L22 (174.4218, -3.175) -> (91.821, -3.175) projected
  arc A39 (88.9, -0.254) -> (91.821, -3.175) centre (91.821, -0.254) ccw projected
  line L23 (149.831, -89.2272) -> (89.9434, -38.9755) projected
  arc A40 (88.9, -36.7379) -> (89.9434, -38.9755) centre (91.821, -36.7379) ccw projected
  line L24 (88.9, -36.7379) -> (88.9, -15.621) projected
  arc A41 (91.821, -12.7) -> (88.9, -15.621) centre (91.821, -15.621) ccw projected
  line L25 (91.821, -12.7) -> (174.1799, -12.7) projected
  arc A42 (177.0893, -15.8819) -> (174.1799, -12.7) centre (174.1799, -15.621) ccw projected
  arc A43 (154.2425, -88.4425) -> (177.0893, -15.8819) centre (0, 0) ccw projected
  arc A44 (149.831, -89.2272) -> (154.2425, -88.4425) centre (151.7086, -86.9895) ccw projected
  circle A45 centre (221.404, -95.9477) radius 3.3782 projected
  circle A46 centre (239.2356, 31.496) radius 3.3782 projected
  circle A47 centre (223.7295, 90.3926) radius 3.3782 projected
  circle A48 centre (239.2356, -31.496) radius 3.3782 projected
  arc A49 (-99.4903, -84.728) -> (-104.0551, -66.155) centre (-101.7058, -75.4251) ccw projected
  arc A50 (-99.6119, -84.758) -> (-99.4903, -84.728) centre (-101.8395, -75.4579) ccw projected
  arc A51 (-99.7334, -84.7881) -> (-99.6119, -84.758) centre (-101.9731, -75.491) ccw projected
  arc A52 (-99.8547, -84.8183) -> (-99.7334, -84.7881) centre (-102.1066, -75.5241) ccw projected
  arc A53 (-104.4917, -66.2632) -> (-99.8547, -84.8183) centre (-102.2399, -75.5574) ccw projected
  arc A54 (-104.3463, -66.227) -> (-104.4917, -66.2632) centre (-102.1066, -75.5241) ccw projected
  arc A55 (-104.2008, -66.1909) -> (-104.3463, -66.227) centre (-101.9731, -75.491) ccw projected
  arc A56 (-104.0551, -66.155) -> (-104.2008, -66.1909) centre (-101.8395, -75.4579) ccw projected
  circle A57 centre (-80.2428, -88.2574) radius 2.4892 projected
  circle A58 centre (-101.8395, -100.8579) radius 2.4892 projected
  circle A59 centre (-93.0185, -51.5569) radius 2.4892 projected
  circle A60 centre (-118.4334, -56.0666) radius 2.4892 projected
  circle A61 centre (-93.2858, -99.3592) radius 2.4892 projected
  circle A62 centre (-110.6604, -51.6228) radius 2.4892 projected
  circle A63 centre (-124.2369, -62.8574) radius 2.4892 projected
  circle A64 centre (-101.8395, -50.0579) radius 2.4892 projected
  circle A65 centre (-110.3931, -99.2933) radius 2.4892 projected
  circle A66 centre (-85.7798, -94.9817) radius 2.4892 projected
  arc A67 (-177.4857, -133.2108) -> (-183.7867, -151.2692) centre (-180.6362, -142.24) ccw projected
  arc A68 (-183.3071, -151.4366) -> (-177.0061, -133.3781) centre (-180.1566, -142.4074) ccw projected
  circle A69 centre (-193.0957, -164.2646) radius 2.4892 projected
  circle A70 centre (-180.6733, -167.7222) radius 2.4892 projected
  circle A71 centre (-168.1768, -164.3742) radius 2.4892 projected
  circle A72 centre (-173.4354, -117.9041) radius 2.4892 projected
  circle A73 centre (-186.8225, -117.6771) radius 2.4892 projected
  circle A74 centre (-193.0957, -120.1058) radius 2.4892 projected
  circle A75 centre (-180.1195, -116.9252) radius 2.4892 projected
  circle A76 centre (-167.2175, -120.5501) radius 2.4892 projected
  circle A77 centre (-174.2102, -166.8866) radius 2.4892 projected
  circle A78 centre (-187.1176, -166.8269) radius 2.4892 projected
  circle A79 centre (-76.4174, -178.6042) radius 13.335 projected
  line L26 (-85.3603, 16.259) -> (-85.3603, 6.734) projected
  arc A80 (-90.1228, 1.9715) -> (-85.3603, 6.734) centre (-90.1228, 6.734) ccw projected
  line L27 (-90.1228, 1.9715) -> (-121.8728, 1.9715) projected
  arc A81 (-126.6353, 6.734) -> (-121.8728, 1.9715) centre (-121.8728, 6.734) ccw projected
  line L28 (-126.6353, 6.734) -> (-126.6353, 16.259) projected
  line L29 (-126.6353, 16.259) -> (-132.3503, 16.259) projected
  arc A82 (-132.3503, 22.609) -> (-132.3503, 16.259) centre (-132.3503, 19.434) ccw projected
  line L30 (-132.3503, 22.609) -> (-126.6353, 22.609) projected
  line L31 (-126.6353, 22.609) -> (-126.6353, 32.134) projected
  arc A83 (-121.8728, 36.8965) -> (-126.6353, 32.134) centre (-121.8728, 32.134) ccw projected
  line L32 (-121.8728, 36.8965) -> (-90.1228, 36.8965) projected
  arc A84 (-85.3603, 32.134) -> (-90.1228, 36.8965) centre (-90.1228, 32.134) ccw projected
  line L33 (-85.3603, 32.134) -> (-85.3603, 22.609) projected
  line L34 (-85.3603, 22.609) -> (-79.6453, 22.609) projected
  arc A85 (-79.6453, 16.259) -> (-79.6453, 22.609) centre (-79.6453, 19.434) ccw projected
  line L35 (-79.6453, 16.259) -> (-85.3603, 16.259) projected
  circle A86 centre (-58.8554, 19.434) radius 2.4892 projected
  line L36 (-112.3478, -13.7765) -> (-99.6478, -13.7765) projected
  arc A87 (-99.6478, -18.8819) -> (-99.6478, -13.7765) centre (-99.6478, -16.3292) ccw projected
  line L37 (-99.6478, -18.8819) -> (-112.3478, -18.8819) projected
  arc A88 (-112.3478, -13.7765) -> (-112.3478, -18.8819) centre (-112.3478, -16.3292) ccw projected
  line L38 (-199.482, -255.599) -> (149.8274, -255.599) projected
  line L39 (194.4526, -163.563) -> (149.8274, -255.599) projected
  arc A89 (194.8736, -162.9119) -> (194.4526, -163.563) centre (197.3095, -164.9483) ccw projected
  arc A90 (194.8736, -162.9119) -> (235.5329, 95.0804) centre (0, 0) ccw projected
  arc A91 (235.5329, 95.0804) -> (218.389, 101.8364) centre (223.7562, 90.3263) ccw projected
  line L40 (218.389, 101.8364) -> (173.6183, 80.9596) projected
  arc A92 (152.1493, 76.2) -> (173.6183, 80.9596) centre (152.1493, 127) ccw projected
  line L41 (152.1493, 76.2) -> (-101.6, 76.2) projected
  line L42 (-101.6, 76.2) -> (-117.9165, 59.8835) projected
  line L43 (-117.9165, 59.8835) -> (-80.5978, 59.8835) projected
  arc A93 (-80.5978, 54.7781) -> (-80.5978, 59.8835) centre (-80.5978, 57.3308) ccw projected
  line L44 (-80.5978, 54.7781) -> (-123.0219, 54.7781) projected
  line L45 (-123.0219, 54.7781) -> (-199.482, -21.682) projected
  line L46 (-199.482, -21.682) -> (-199.482, -255.599) projected
  line L47 (-177.4857, -133.2108) -> (-177.0061, -133.3781) projected
  line L48 (-183.3071, -151.4366) -> (-183.7867, -151.2692) projected
  point P0 (-59.782, 63.5)
  point P1 (-8.982, 63.5)
  point P2 (67.218, 63.5)
  point P3 (143.418, 63.5)
  point P4 (-186.782, -242.899)
  point P5 (-186.782, -179.399)
  point P6 (-186.782, -39.699)
  point P7 (-148.682, -242.899)
  point P8 (-148.682, -179.399)
  point P9 (-148.682, -39.699)
  point P10 (-116.932, -242.899)
  point P11 (-116.932, -179.399)
  point P12 (-116.932, -39.699)
  dimension "d518" = 12.7
  dimension "d519" = 12.7
  dimension "d520" = 12.7
  dimension "d521" = 76.2
  dimension "d522" = 215.9
  dimension "d523" = 139.7
  dimension "d524" = 50.8
  dimension "d525" = 76.2
  dimension "d526" = 76.2
  dimension "d534" = 38.1
  dimension "d535" = 31.75
  dimension "d870" = 0
  constraints: 8 horizontal alignment, 6 vertical alignment
  measures "d518" distance from line of L0 point (143.418, 63.5)
  measures "d519" distance from line of point (-186.782, -242.899) L2
  measures "d520" distance from line of point (-186.782, -242.899) L1
  measures "d521" distance from line of point (-186.782, -179.399) L1
  measures "d522" distance from line of point (-186.782, -39.699) L1
  measures "d523" distance from line of point (-59.782, 63.5) L2
  measures "d524" distance of point (-8.982, 63.5) point (-59.782, 63.5)
  measures "d525" distance of point (67.218, 63.5) point (-8.982, 63.5)
  measures "d526" distance of point (143.418, 63.5) point (67.218, 63.5)
  measures "d534" distance of point (-148.682, -242.899) point (-186.782, -242.899)
  measures "d535" distance of point (-148.682, -242.899) point (-116.932, -242.899)
  measures "d870" vertical distance of point (-148.682, -39.699) point (-116.932, -39.699)
hole "MountingHoles" at (0, 63.5, 59.782) at (0, 63.5, 8.982) at (0, 63.5, -67.218) at (0, 63.5, -143.418) at (0, -242.899, 186.782) at (0, -179.399, 186.782) at (0, -39.699, 186.782) at (0, -39.699, 148.682) at (0, -179.399, 148.682) at (0, -39.699, 116.932) at (0, -179.399, 116.932) at (0, -242.899, 148.682) at (0, -242.899, 116.932) direction (-1, 0, 0) diameter 5.1054 end through all clearance for "Flat Head Machine Screw (82)" size "#10" standard "Ansi Unified Screw Threads"
sketch "Sketch33" plane through (0, 0, 0) normal (1, 0, 0) x (0, 0, -1)
  circle A0 centre (0, 0) radius 22.225 construction
  line L0 (0, 0) -> (22.225, 0) construction
  line L1 (0, -0.9595) -> (22.2043, -0.9595) construction
  point P0 (11.1125, 19.2474)
  point P1 (-11.1125, 19.2474)
  point P2 (-22.225, 0)
  point P3 (-11.1125, -19.2474)
  point P4 (11.1125, -19.2474)
  dimension "d540" = 0
  dimension "d543" = 360
  dimension "d545" = 44.45
  constraints: 4 end point, 2 point on circle, 1 centre point, 1 coincident, 1 horizontal, 7 other
  measures "d540" angle of L0 L1
  measures "d545" diameter of A0
hole "HoodPivotHoles" at (0, 0, -22.225) at (0, 19.2474, -11.1125) at (0, 19.2474, 11.1125) at (0, 0, 22.225) at (0, -19.2474, 11.1125) at (0, -19.2474, -11.1125) direction (-1, 0, 0) diameter 4.4958 end through all clearance for "Flat Head Machine Screw (82)" size "#8" standard "Ansi Unified Screw Threads"